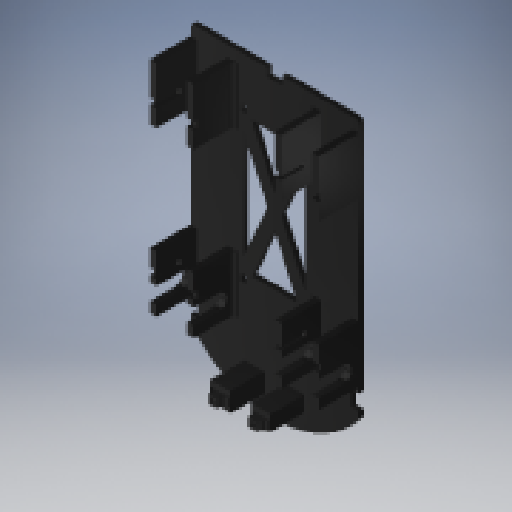
# Autodesk Inventor part: BASE
Saved by Autodesk Inventor 2025.1 (Build 291241020, 241B)
## iProperties
Created: 2024-12-26
Part Number: BASE
Material: Genérico
Document SubType Name: Modeling
Designer: 53433618895
Density: 1 g/cm^3
Appearance: Suave - Preto
Author: 53433618895
Autodesk Inventor part; units mm, degrees
ref_plane "YZ Plane" through (0, 0, 0) normal (1, 0, 0) x (0, 1, 0)
ref_plane "XZ Plane" through (0, 0, 0) normal (0, 1, 0) x (-1, 0, 0)
ref_plane "XY Plane" through (0, 0, 0) normal (0, 0, 1) x (1, 0, 0)
sketch "Esboço1" plane through (0, 0, 0) normal (0, 0, 1) x (1, 0, 0)
  arc A0 (-52.15, -67.3833) -> (52.15, -67.3833) centre (0, -27.4378) ccw
  line L0 (52.15, -67.3833) -> (52.15, 91.1285)
  line L1 (50.15, 93.1285) -> (-50.15, 93.1285)
  line L2 (-52.15, 91.1285) -> (-52.15, -67.3833)
  arc A1 (-50.15, 93.1285) -> (-52.15, 91.1285) centre (-50.15, 91.1285) ccw
  arc A2 (52.15, 91.1285) -> (50.15, 93.1285) centre (50.15, 91.1285) ccw
  point P0 (0, 0)
  point P1 (49.15, -65.3715)
  dimension "d2" = 104.3
  dimension "d147" = 2
  constraints: 8 point on circle, 6 end point, 3 centre point, 2 tangent, 1 horizontal, 1 vertical, 1 other
  measures "d2" distance between parallel lines of L2 L0
  measures "d147" radius of A2
extrude "Extrusão1" add sketch "Esboço1" along normal blind 3
sketch "Esboço2" plane through (0, 0, 3) normal (0, 0, 1) x (1, 0, 0)
  line L0 (-52.15, 91.1285) -> (-52.15, -67.3833) projected
  line L1 (-48.15, 86.1285) -> (-52.15, 86.1285)
  line L2 (-52.15, 86.1285) -> (-52.15, 51.1285)
  line L3 (-52.15, 51.1285) -> (-48.15, 51.1285)
  line L4 (-48.15, 51.1285) -> (-48.15, 86.1285)
  line L5 (-29.15, 86.1285) -> (-25.15, 86.1285)
  line L6 (-25.15, 86.1285) -> (-25.15, 51.1285)
  line L7 (-25.15, 51.1285) -> (-29.15, 51.1285)
  line L8 (-29.15, 51.1285) -> (-29.15, 86.1285)
  line L9 (50.15, 93.1285) -> (-50.15, 93.1285) projected
  line L10 (25.15, 51.1285) -> (29.15, 51.1285)
  line L11 (29.15, 51.1285) -> (29.15, 86.1285)
  line L12 (48.15, 51.1285) -> (48.15, 86.1285)
  line L13 (52.15, 86.1285) -> (52.15, 51.1285)
  line L14 (48.15, 86.1285) -> (52.15, 86.1285)
  line L15 (25.15, 86.1285) -> (25.15, 51.1285)
  line L16 (29.15, 86.1285) -> (25.15, 86.1285)
  line L17 (-52.15, -49.8715) -> (-48.15, -49.8715)
  line L18 (-48.15, -49.8715) -> (-48.15, -14.8715)
  line L19 (-29.15, -49.8715) -> (-29.15, -14.8715)
  line L20 (-25.15, -14.8715) -> (-25.15, -49.8715)
  line L21 (-29.15, -14.8715) -> (-25.15, -14.8715)
  line L22 (-52.15, -14.8715) -> (-52.15, -49.8715)
  line L23 (-48.15, -14.8715) -> (-52.15, -14.8715)
  line L24 (25.15, -49.8715) -> (29.15, -49.8715)
  line L25 (29.15, -49.8715) -> (29.15, -14.8715)
  line L26 (48.15, -49.8715) -> (48.15, -14.8715)
  line L27 (52.15, -14.8715) -> (52.15, -49.8715)
  line L28 (48.15, -14.8715) -> (52.15, -14.8715)
  line L29 (25.15, -14.8715) -> (25.15, -49.8715)
  line L30 (29.15, -14.8715) -> (25.15, -14.8715)
  line L31 (48.15, 51.1285) -> (52.15, 51.1285)
  line L32 (48.15, -49.8715) -> (52.15, -49.8715)
  line L33 (-29.15, -49.8715) -> (-25.15, -49.8715)
  point P0 (0, 0)
  point P1 (-52.15, -55.7715)
  point P2 (-4.8, 93.1285)
  point P3 (-52.15, -14.8715)
  point P4 (-52.15, -49.8715)
  point P5 (-52.15, -40.7822)
  point P6 (-52.15, -50.9822)
  point P7 (17.852, 93.1285)
  point P8 (7.652, 93.1285)
  point P9 (-52.15, -40.7822)
  dimension "d6" = 4
  dimension "d7" = 4
  dimension "d8" = 35
  dimension "d9" = 7
  dimension "d10" = 19
  dimension "d17" = 77.3
  dimension "d20" = 101
  constraints: 64 end point, 9 point on line, 6 equal length, 4 horizontal, 2 perpendicular, 1 vertical, 45 other
  measures "d6" distance of L2.end L3.end
  measures "d7" distance of L6.end L7.end
  measures "d8" distance of L5.end L6.end
  measures "d9" distance between parallel lines of L9 L5
  measures "d10" distance between parallel lines of L8 L4
  measures "d17" distance of L2.end L10.start
  measures "d20" distance of L2.end L17.start
extrude "Extrusão2" add sketch "Esboço2" along normal blind 25
sketch "Esboço4" plane through (-52.15, -35.7715, 0) normal (-1, 0, 0) x (0, 0, 1)
  line L0 (3, 121.9) -> (28, 121.9) projected
  line L1 (28, 20.9) -> (28, 86.9) projected
  line L2 (3, 86.9) -> (28, 86.9) projected
  line L3 (28, 105.6) -> (12.6, 105.6)
  line L4 (28, 115.6) -> (12.6, 115.6)
  arc A0 (12.6, 115.6) -> (12.6, 105.6) centre (12.6, 110.6) ccw
  circle A1 centre (15.7, 99.6) radius 3 construction
  line L5 (28, 97.6) -> (28, 101.6)
  line L6 (28, 14.6) -> (28, 4.6)
  line L7 (28, 0.6) -> (28, -3.4)
  line L8 (28, -14.1) -> (28, 20.9) projected
  line L9 (28, 86.9) -> (28, 20.9)
  line L10 (28, 53.9) -> (-7.479, 53.9)
  line L11 (28, 2.2) -> (12.6, 2.2)
  line L12 (28, -7.8) -> (12.6, -7.8)
  arc A2 (12.6, 2.2) -> (12.6, -7.8) centre (12.6, -2.8) ccw
  line L13 (28, 115.6) -> (28, 105.6)
  line L14 (28, 86.9) -> (28, 121.9) projected
  point P0 (0, 35.7715)
  point P1 (7.6, 110.6)
  point P2 (25, 99.6)
  point P3 (28, -7.8)
  dimension "d24" = 10
  dimension "d25" = 20.4
  dimension "d26" = 6.3
  dimension "d27" = 6
  dimension "d28" = 12.3
  dimension "d29" = 6
  dimension "d33" = 0
  dimension "d36" = 101
  constraints: 20 end point, 5 point on circle, 5 symmetric about line, 3 centre point, 3 collinear, 3 horizontal, 3 point on line, 2 tangent, 1 midpoint, 1 other
  measures "d24" distance between parallel lines of L3 L4
  measures "d25" distance from line of L1 point (7.6, 110.6)
  measures "d26" distance between parallel lines of L0 L4
  measures "d27" diameter of A1
  measures "d28" distance from line of L1 A1.centre
  measures "d29" distance from line of L3 A1.centre
  measures "d33" vertical distance of A1.centre point (25, 99.6)
  measures "d36" distance of L4.start L6.start
extrude "Extrusão4" cut sketch "Esboço4" against normal through all
sketch "Esboço5" plane through (0, 0, 28) normal (0, 0, 1) x (1, 0, 0)
  line L0 (-48.15, 65.8285) -> (-48.15, 61.8285) projected
  line L1 (25.15, 65.8285) -> (-48.15, 65.8285) projected
  line L2 (-48.15, 61.8285) -> (25.15, 61.8285) projected
  line L3 (-48.15, 65.8285) -> (-50.15, 65.8285)
  line L4 (-50.15, 65.8285) -> (-50.15, 61.8285)
  line L5 (-50.15, 61.8285) -> (-48.15, 61.8285)
  line L6 (-48.15, 61.8285) -> (-48.15, 65.8285)
  line L7 (-50.15, -25.5715) -> (-50.15, -29.5715)
  line L8 (-48.15, -25.5715) -> (-50.15, -25.5715)
  line L9 (-48.15, -29.5715) -> (-48.15, -25.5715)
  line L10 (-50.15, -29.5715) -> (-48.15, -29.5715)
  line L11 (-29.15, 65.8285) -> (-29.15, 61.8285)
  line L12 (-27.15, 65.8285) -> (-29.15, 65.8285)
  line L13 (-27.15, 61.8285) -> (-27.15, 65.8285)
  line L14 (-29.15, 61.8285) -> (-27.15, 61.8285)
  line L15 (-29.15, -25.5715) -> (-29.15, -29.5715)
  line L16 (-27.15, -25.5715) -> (-29.15, -25.5715)
  line L17 (-27.15, -29.5715) -> (-27.15, -25.5715)
  line L18 (-29.15, -29.5715) -> (-27.15, -29.5715)
  line L19 (48.15, 61.8285) -> (50.15, 61.8285)
  line L20 (29.15, 65.8285) -> (27.15, 65.8285)
  line L21 (27.15, 65.8285) -> (27.15, 61.8285)
  line L22 (29.15, 61.8285) -> (29.15, 65.8285)
  line L23 (48.15, 65.8285) -> (48.15, 61.8285)
  line L24 (50.15, 61.8285) -> (50.15, 65.8285)
  line L25 (50.15, 65.8285) -> (48.15, 65.8285)
  line L26 (27.15, 61.8285) -> (29.15, 61.8285)
  line L27 (50.15, -25.5715) -> (48.15, -25.5715)
  line L28 (50.15, -29.5715) -> (50.15, -25.5715)
  line L29 (48.15, -29.5715) -> (50.15, -29.5715)
  line L30 (48.15, -25.5715) -> (48.15, -29.5715)
  line L31 (29.15, -25.5715) -> (27.15, -25.5715)
  line L32 (29.15, -29.5715) -> (29.15, -25.5715)
  line L33 (27.15, -25.5715) -> (27.15, -29.5715)
  line L34 (27.15, -29.5715) -> (29.15, -29.5715)
  point P0 (0, 0)
  point P1 (-52.15, 65.8285)
  point P2 (-52.15, 61.8285)
  dimension "d43" = 2
  dimension "d46" = 91.4
  dimension "d49" = 21
  dimension "d54" = 77.3
  constraints: 64 end point, 3 horizontal, 2 parallel, 1 perpendicular, 1 point on line, 1 vertical, 59 other
  measures "d43" distance of L5.end L4.end
  measures "d46" distance of L3.end L7.start
  measures "d49" distance of L3.end L11.start
  measures "d54" distance of L0.start L20.start
extrude "Extrusão5" cut sketch "Esboço5" against normal blind 13.5 contours L0 L5 L4 L3 | L1 L13 L2 L11 | L8 L9 L10 L7 | L16 L17 L18 L15 | L23 L25 L24 L19 | L22 L26 L21 L20 | L28 L29 L30 L27 | L32 L34 L33 L31
fillet "Arredondamento1" radius 3 4 edges at (-25.15, -32.3715, 3) (-25.15, 68.6285, 3) (25.15, 68.6285, 3) (25.15, -32.3715, 3)
sketch "Esboço8" plane through (-48.15, -49.8715, 3) normal (1, 0, 0) x (0, 0, -1)
  line L0 (-11.5, 24.3) -> (-11.5, 20.3) projected
  line L1 (-25, 24.3) -> (-11.5, 24.3) projected
  circle A0 centre (-11.5, 22.3) radius 2
  point P0 (3, 49.8715)
  point P1 (-11.5, 20.3)
  constraints: 1 midpoint, 3 other
extrude "Extrusão7" cut sketch "Esboço8" along normal blind 21 and the other way blind 2 contours A0 L0 picked at (-10.9788, 22.7157)
sketch "Esboço9" plane through (-48.15, 51.1285, 3) normal (1, 0, 0) x (0, 0, -1)
  line L0 (-11.5, 14.7) -> (-11.5, 10.7) projected
  circle A0 centre (-11.5, 12.7) radius 2
  point P0 (3, -51.1285)
  constraints: 1 midpoint, 3 other
extrude "Extrusão8" cut sketch "Esboço9" along normal blind 21 and the other way blind 2 contours A0 L0 picked at (-10.8304, 13.0989)
sketch "Esboço10" plane through (29.15, 51.1285, 3) normal (1, 0, 0) x (0, 0, -1)
  line L0 (-11.5, 14.7) -> (-11.5, 10.7) projected
  circle A0 centre (-11.5, 12.7) radius 2
  point P0 (3, -51.1285)
  constraints: 1 midpoint, 3 other
extrude "Extrusão9" cut sketch "Esboço10" along normal blind 21 and the other way blind 2 contours A0 L0 picked at (-10.8304, 13.0989)
sketch "Esboço11" plane through (29.15, -49.8715, 3) normal (1, 0, 0) x (0, 0, -1)
  line L0 (-11.5, 24.3) -> (-11.5, 20.3) projected
  circle A0 centre (-11.5, 22.3) radius 2
  point P0 (3, 49.8715)
  constraints: 1 midpoint, 3 other
extrude "Extrusão10" cut sketch "Esboço11" along normal blind 21 and the other way blind 2 contours A0 L0 picked at (-10.9788, 22.7157)
sketch "Esboço12" plane through (0, 0, 3) normal (0, 0, 1) x (1, 0, 0)
  line L0 (0, 0) -> (0, -42.6035)
  circle A0 centre (-12.5, -76.9378) radius 1.25
  line L1 (-15, -79.4378) -> (-10, -79.4378)
  line L2 (-10, -79.4378) -> (-10, -74.4378)
  line L3 (-10, -74.4378) -> (-15, -74.4378)
  line L4 (-15, -74.4378) -> (-15, -79.4378)
  line L5 (-15, -79.4378) -> (-10, -74.4378) construction
  line L6 (-10, -79.4378) -> (-15, -74.4378) construction
  circle A1 centre (12.5, -76.9378) radius 1.25
  line L7 (15, -79.4378) -> (10, -79.4378)
  line L8 (10, -79.4378) -> (10, -74.4378)
  line L9 (10, -74.4378) -> (15, -74.4378)
  line L10 (15, -74.4378) -> (15, -79.4378)
  line L11 (15, -79.4378) -> (10, -74.4378) construction
  line L12 (10, -79.4378) -> (15, -74.4378) construction
  point P0 (-38.6877, -67.9255)
  point P1 (38.6877, -67.9255)
  point P2 (0, -27.4378)
  dimension "d96" = 2.5
  dimension "d97" = 5
  dimension "d98" = 52
  dimension "d99" = 25
  constraints: 26 end point, 5 symmetric about line, 2 centre point, 2 horizontal, 2 midpoint, 2 parallel, 2 perpendicular, 1 vertical, 1 other
  measures "d96" diameter of A0
  measures "d97" distance of L3.end L2.end
  measures "d98" distance from line of point (0, -27.438) L1
  measures "d99" diameter of A0.centre L0
extrude "Extrusão11" add sketch "Esboço12" along normal blind 26
sketch "Esboço13" plane through (0, 0, 3) normal (0, 0, 1) x (1, 0, 0)
  line L0 (6.5, -82.9378) -> (18.5, -82.9378)
  line L1 (18.5, -82.9378) -> (18.5, -70.9378)
  line L2 (18.5, -70.9378) -> (6.5, -70.9378)
  line L3 (6.5, -70.9378) -> (6.5, -82.9378)
  circle A0 centre (12.5, -76.9378) radius 1.25 projected
  line L4 (6.5, -82.9378) -> (18.5, -70.9378) construction
  line L5 (18.5, -82.9378) -> (6.5, -70.9378) construction
  line L6 (-18.5, -82.9378) -> (-6.5, -82.9378)
  line L7 (-6.5, -82.9378) -> (-6.5, -70.9378)
  line L8 (-6.5, -70.9378) -> (-18.5, -70.9378)
  line L9 (-18.5, -70.9378) -> (-18.5, -82.9378)
  circle A1 centre (-12.5, -76.9378) radius 1.25 projected
  line L10 (-18.5, -82.9378) -> (-6.5, -70.9378) construction
  line L11 (-6.5, -82.9378) -> (-18.5, -70.9378) construction
  arc A2 (-38.6877, -67.9255) -> (38.6877, -67.9255) centre (0, -27.4378) ccw projected
  point P0 (0, 0)
  point P1 (7.4666, -82.9378)
  point P2 (18.5, -80.2937)
  point P3 (-18.5, -80.2937)
  point P4 (-7.4666, -82.9378)
  dimension "d102" = 12
  constraints: 24 end point, 5 perpendicular, 4 midpoint, 4 parallel, 2 horizontal
  measures "d102" distance of L2.end L1.end
extrude "Extrusão12" add sketch "Esboço13" along normal blind 21 contours L3 L2 L1 A2 L0 | A2 L9 L8 L7 L6
fillet "Arredondamento2" radius 6 4 edges at (15, -76.9378, 24) (10, -76.9378, 24) (-15, -76.9378, 24) (-10, -76.9378, 24)
sketch "Esboço16" plane through (0, 0, 3) normal (0, 0, 1) x (1, 0, 0)
  line L0 (22.15, 61.8285) -> (19.85, 61.8285) construction
  line L1 (20.999, 61.8285) -> (-21.15, 61.8285) construction
  line L2 (-21.15, 61.8285) -> (-21.15, -25.5715) construction
  line L3 (-21.15, -25.5715) -> (20.999, -25.5715) construction
  line L4 (20.999, -25.5715) -> (20.999, 61.8285) construction
  line L5 (13.999, 59.8285) -> (-14.15, 59.8285)
  line L6 (-19.15, 54.8285) -> (-19.15, -18.5715)
  line L7 (-14.15, -23.5715) -> (13.999, -23.5715)
  line L8 (18.999, -18.5715) -> (18.999, 54.8285)
  arc A0 (18.999, 54.8285) -> (13.999, 59.8285) centre (13.999, 54.8285) ccw
  arc A1 (-14.15, 59.8285) -> (-19.15, 54.8285) centre (-14.15, 54.8285) ccw
  arc A2 (-19.15, -18.5715) -> (-14.15, -23.5715) centre (-14.15, -18.5715) ccw
  arc A3 (13.999, -23.5715) -> (18.999, -18.5715) centre (13.999, -18.5715) ccw
  line L9 (-17.6855, 58.364) -> (17.5345, -22.1071) construction
  line L10 (17.5345, 58.364) -> (-17.6855, -22.1071) construction
  line L11 (21.1989, 56.7602) -> (-14.0211, -23.7109)
  line L12 (13.8701, 59.9678) -> (-21.3499, -20.5033)
  line L13 (-21.3499, 56.7602) -> (13.8701, -23.7109)
  line L14 (-14.0211, 59.9678) -> (21.1989, -20.5033)
  point P0 (0, 0)
  point P1 (-4.4418, 18.1285)
  point P2 (-19.15, 51.7338)
  point P3 (-19.15, -15.4769)
  point P4 (13.8092, -23.5715)
  point P5 (-0.0755, 8.1522)
  point P6 (-13.9602, -23.5715)
  point P7 (4.2908, 18.1285)
  point P8 (18.999, -15.4769)
  point P9 (18.999, 51.7338)
  point P10 (-13.9602, 59.8285)
  point P11 (-0.0755, 28.1047)
  point P12 (13.8092, 59.8285)
  dimension "d139" = 2
  dimension "d140" = 5
  dimension "d141" = 4
  dimension "d142" = 4
  dimension "d143" = 4
  dimension "d144" = 4
  constraints: 28 end point, 12 point on circle, 8 parallel, 8 tangent, 4 centre point, 3 equal radius, 2 perpendicular, 1 horizontal, 3 other
  measures "d139" distance between parallel lines of L4 L8
  measures "d140" radius of A0
  measures "d141" distance between parallel lines of L10 L11
  measures "d142" distance between parallel lines of L10 L12
  measures "d143" distance between parallel lines of L9 L13
  measures "d144" distance between parallel lines of L9 L14
extrude "Extrusão15" cut sketch "Esboço16" against normal blind 10 contours L12 L14 L5 | L8 L14 L11 | L12 L6 L13 | L13 L7 L11
sketch "Esboço17" plane through (0, 0, 3) normal (0, 0, 1) x (1, 0, 0)
  line L0 (-47.15, -53.2715) -> (-47.15, -62.8715) projected
  line L1 (-50.65, -62.8715) -> (-47.15, -62.8715) projected
  line L2 (-50.65, -53.2715) -> (-47.15, -53.2715) projected
  line L3 (47.15, -62.8715) -> (47.15, -53.2715) projected
  line L4 (50.65, -62.8715) -> (47.15, -62.8715) projected
  line L5 (50.65, -53.2715) -> (47.15, -53.2715) projected
  line L6 (-4.8, 91.6285) -> (-4.8, 88.1285) projected
  line L7 (4.8, 88.1285) -> (-4.8, 88.1285) projected
  line L8 (4.8, 91.6285) -> (4.8, 88.1285) projected
  line L9 (50.15, 93.1285) -> (-50.15, 93.1285) projected
  line L10 (-52.15, -49.8715) -> (-52.15, -67.3833) projected
  line L11 (52.15, -67.3833) -> (52.15, -49.8715) projected
  line L12 (-4.8, 91.6285) -> (-4.8, 93.1285)
  line L13 (4.8, 91.6285) -> (4.8, 93.1285)
  line L14 (50.65, -62.8715) -> (52.15, -62.8715)
  line L15 (50.65, -53.2715) -> (52.15, -53.2715)
  line L16 (-50.65, -62.8715) -> (-52.15, -62.8715)
  line L17 (-50.65, -53.2715) -> (-52.15, -53.2715)
  point P0 (0, 0)
  constraints: 12 end point, 8 point on line, 4 perpendicular
extrude "Extrusão16" cut sketch "Esboço17" against normal through all
fillet "Arredondamento3" radius 2 11 edges at (13.8092, 59.8285, 1.5) (-0.0755, 28.1047, 1.5) (18.999, -15.4769, 1.5) (18.999, 51.7338, 1.5) (-19.15, 51.7338, 1.5) (-4.4418, 18.1285, 1.5) (4.2908, 18.1285, 1.5) (-13.9602, -23.5715, 1.5) (-0.0755, 8.1522, 1.5) (-19.15, -15.4769, 1.5) (-13.9602, 59.8285, 1.5)
fillet "Arredondamento4" radius 2 1 edges at (13.8092, -23.5715, 1.5)
equation "\"d6\" = d7"
